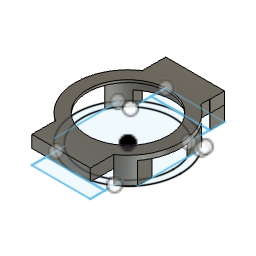
g-shock (Autodesk Fusion 360 design; units mm, degrees)
Autodesk Fusion 360 part; units mm, degrees
sketch "Sketch1" plane through (0, 0, 0) normal (0, 0, 1) x (1, 0, 0)
  circle A0 centre (0, 0) radius 18.5
  circle A1 centre (0, 0) radius 21.5
  line L0 (0, 21.5) -> (12, 21.5)
  line L1 (0, 21.5) -> (-12, 21.5)
  line L2 (-12, 21.5) -> (-12, 17.8396)
  line L3 (12, 21.5) -> (12, 17.8396)
  line L4 (-12, 21.5) -> (-12, 27.5)
  line L5 (-12, 21.5) -> (12.1388, 21.5)
  line L6 (12.1388, 21.5) -> (12.1388, 27.5)
  line L7 (12.1388, 27.5) -> (-12, 27.5)
  line L8 (0, -21.5) -> (12, -21.5)
  line L9 (12, -21.5) -> (-12, -21.5)
  line L10 (-12, -21.5) -> (-12, -27.5)
  line L11 (-12, -27.5) -> (12, -27.5)
  line L12 (12, -27.5) -> (12, -21.5)
  line L13 (-12, -21.5) -> (12, -21.5)
  line L14 (12, -21.5) -> (12, -17.5)
  line L15 (-12, -17.5) -> (-12, -21.5)
  line L16 (17.0336, 12.9751) -> (17.0336, -13.1189)
  line L17 (-16.9608, 12.9009) -> (-16.9608, -13.2129)
  line L18 (-16.9608, 7.3879) -> (-16.9608, 13.2129)
  line L19 (17.0336, 7.2185) -> (17.0336, 14.6093)
  line L20 (-12, -27.5) -> (-12, -14.0801)
  line L21 (12, -27.5) -> (12, -14.0801)
  line L22 (12.1388, 27.5) -> (12, 13)
  line L23 (-12, 27.5) -> (-12, 13)
  dimension "d1" = 37
  dimension "d2" = 43
  dimension "d3" = 12
  dimension "d4" = 12
  dimension "d5" = 6
  dimension "d8" = 24
  dimension "d9" = 6
  dimension "d10" = 24
  dimension "d11" = 4
  dimension "d12" = 7
  dimension "d13" = 7
  constraint coincident A0.centre A1.centre
  constraint concentric A0 A1
  constraint coincident A1 L0.start
  constraint horizontal L0
  constraint parallel L0 L1
  constraint coincident A1 L2.end
  constraint perpendicular L1 L2
  constraint coincident A1 L3.end
  constraint perpendicular L0 L3
  constraint perpendicular L1 L4
  constraint horizontal L5
  constraint vertical L6
  constraint horizontal L7
  constraint coincident A1 L8.start
  constraint horizontal L8
  constraint horizontal L9
  constraint vertical L10
  constraint horizontal L11
  constraint vertical L12
  constraint horizontal L13
  constraint vertical L14
  constraint vertical L15
  constraint coincident A1 L16.end
  constraint vertical L16
  constraint coincident A1 L17.end
  constraint vertical L17
  constraint coincident A0 L18.start
  constraint coincident L17 L18.start
  constraint coincident A1 L18.end
  constraint parallel L17 L18
  constraint coincident A0 L19.start
  constraint coincident L16 L19.start
  constraint parallel L16 L19
  constraint coincident A0 L20.end
  constraint perpendicular L11 L20
  constraint coincident A0 L21.end
  constraint perpendicular L11 L21
  constraint parallel L4 L23
  measures "d1" diameter of A0
  measures "d2" diameter of A1
  measures "d3" distance of L0.start L0.end
  measures "d4" distance of L0.start L1.end
  measures "d5" distance of L1.end L4.end
  measures "d8" distance of L8.end L9.end
  measures "d9" distance of L8.end L11.end
  measures "d10" distance of L9.end L8.end
  measures "d11" distance of L9.end L15.start
  measures "d12" distance of L3.end L16.start
  measures "d13" distance of L2.end L17.start
extrude "Extrude1" add sketch "Sketch1" along normal blind 11 contours A0 A1 L16 L19 L22 | A0 A1 L14 L16 L21 | A0 A1 L22 L23 | A0 A1 L14 L15 L20 L21 | A0 A1 L17 L18 L23 | A0 A1 L15 L17 L20 | A1 L8 L9 L13 L14 L21 | A1 L1 L2 L5 L23 | A1 L0 L3 L5 | L5 L6 L22 | L0 L1 L4 L5 L7 L22 L23 | A1 L9 L13 L15 L20 | L8 L9 L10 L11 L12 L13 L20 L21 makes body 1 at (-15.2167, 10.5216, 7.3333) makes body 2 at (16.2537, -8.8355, 3.6667)
extrude "Extrude2" add sketch "Sketch1" along normal blind 11 contours A0 A1 L16 L19 | A0 A1 L17 L18 bodies 1 2
extrude "Extrude3" cut sketch "Sketch1" along normal blind 9 contours A0 A1 L16 L19 | A0 A1 L17 L18 bodies 1
sketch "Sketch2" plane through (0, 0, 11) normal (0, 0, 1) x (-1, 0, 0)
  arc A0 (12, -17.8396) -> (12, 17.8396) centre (0, 0) ccw
  line L0 (12, 17.8396) -> (12, 27.5)
  line L1 (12, 27.5) -> (-12, 27.5)
  line L2 (-12, 27.5) -> (-12, 17.8396)
  arc A1 (-12, 17.8396) -> (-12, -17.8396) centre (0, 0) ccw
  line L3 (-12, -17.8396) -> (-12, -21.5)
  line L4 (-12, -21.5) -> (-12.1388, -21.5)
  line L5 (-12.1388, -21.5) -> (-12.1388, -27.5)
  line L6 (-12.1388, -27.5) -> (12, -27.5)
  line L7 (12, -27.5) -> (12, -17.8396)
  circle A2 centre (0, 0) radius 18.5
  circle A3 centre (0, 0) radius 16.5
  circle A4 centre (0, 0) radius 18.5
  dimension "d20" = 33
  constraint coincident A0.centre A1.centre
  constraint concentric A3 A4
  measures "d20" diameter of A3
extrude "Extrude4" add sketch "Sketch2" against normal blind 1 contours A2 A4 bodies 1
extrude "Extrude5" cut sketch "Sketch1" along normal blind 6 contours A0 A1 L14 L15 L20 L21 | A1 L8 L9 L13 L14 L21 | A1 L9 L13 L15 L20 | L8 L9 L10 L11 L12 L13 L20 L21 bodies 1
extrude "Extrude6" cut sketch "Sketch1" along normal blind 6 contours A0 A1 L22 L23 | A1 L1 L2 L5 L23 | A1 L0 L3 L5 | L0 L1 L4 L5 L7 L22 L23 bodies 1
